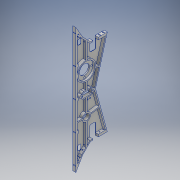
# Autodesk Inventor part: 옆판_왼쪽
Saved by Autodesk Inventor 2017 (Build 210142000, 142)
## iProperties
Part Number: 옆판_왼쪽
Material: 알루미늄 6061
Document SubType Name: Modeling
Designer: minom
Density: 2.7 g/cm^3
Appearance: 알루미늄 - 평지
Mass: 105.833 g
Surface Area: 460.964 cm^2
Volume: 39.1973 cm^3
Author: minom
Autodesk Inventor part; units mm, degrees
(part 1 of 2)
ref_plane "YZ Plane" through (0, 0, 0) normal (1, 0, 0) x (0, 1, 0)
ref_plane "XZ Plane" through (0, 0, 0) normal (0, 1, 0) x (-1, 0, 0)
ref_plane "XY Plane" through (0, 0, 0) normal (0, 0, 1) x (1, 0, 0)
sketch "스케치1" plane through (0, 0, 0) normal (1, 0, 0) x (0, 1, 0)
  line L0 (0, 0) -> (0, -320)
  line L1 (0, -320) -> (0, -270)
  line L2 (0, -270) -> (0, -290)
  line L3 (0, 0) -> (0, -50)
  line L4 (0, -50) -> (0, -30)
  line L5 (0, -30) -> (60, -30)
  line L6 (80, -50) -> (80, -270)
  line L7 (80, -270) -> (0, -270)
  line L8 (0, -290) -> (80, -290)
  line L9 (0, -50) -> (80, -50)
  line L10 (0, 0) -> (17.3205, -30)
  line L11 (0, 0) -> (34.641, 0) construction
  line L12 (17.3205, -30) -> (37.3205, -50)
  line L13 (17.3205, -30) -> (45.6048, -30) construction
  line L14 (0, -320) -> (17.3205, -290)
  line L15 (0, -320) -> (34.641, -320) construction
  line L16 (17.3205, -290) -> (37.3205, -270)
  line L17 (17.3205, -290) -> (45.6048, -290) construction
  dimension "d0" = 320
  dimension "d1" = 50
  dimension "d2" = 50
  dimension "d3" = 20
  dimension "d4" = 60
  dimension "d5" = 60
  dimension "d6" = 45
  dimension "d7" = 60
  dimension "d8" = 45
  dimension "d37" = 80
  constraints: 36 end point, 9 point on line, 4 equal length, 4 horizontal, 4 perpendicular, 1 parallel, 1 vertical
  measures "d0" distance of L0.start L0.end
  measures "d1" distance of L0.end L1.end
  measures "d2" distance of L0.start L3.end
  measures "d3" distance of L3.end L4.end
  measures "d4" distance of L4.end L5.end
  measures "d5" angle of L10 L11
  measures "d6" angle of L12 L13
  measures "d7" angle of L15 L14
  measures "d8" angle of L17 L16
  measures "d37" distance between parallel lines of L0 L6
extrude "돌출1" add sketch "스케치1" along normal blind 8
sketch "스케치2" plane through (8, 0, 0) normal (1, 0, 0) x (0, 0, -1)
  line L0 (270, 37.3205) -> (270, 80) projected
  line L1 (270, 80) -> (50, 80) projected
  line L2 (109, 80) -> (109, 27)
  circle A0 centre (109, 27) radius 21.25
  line L3 (50, 80) -> (50, 37.3205) projected
  line L4 (0, 0) -> (320, 0) projected
  dimension "d13" = 42.5
  dimension "d16" = 59
  dimension "d149" = 27
  constraints: 2 end point, 1 centre point, 1 coincident, 1 point on line
  measures "d13" diameter of A0
  measures "d16" distance between parallel lines of L2 L3
  measures "d149" distance from line of L4 L2.end
extrude "돌출2" cut sketch "스케치2" against normal blind 5
sketch "스케치3" plane through (3, 27, -109) normal (1, 0, 0) x (0, 0, -1)
  circle A0 centre (0, 0) radius 21.25 projected
  line L0 (-59, 10.3205) -> (-79, -9.6795) projected
  line L1 (-79, -9.6795) -> (-109, -27) projected
  line L2 (-109, -27) -> (211, -27) projected
  line L3 (211, -27) -> (181, -9.6795) projected
  line L4 (181, -9.6795) -> (161, 10.3205) projected
  line L5 (161, 10.3205) -> (161, 53) projected
  line L6 (161, 53) -> (-59, 53) projected
  line L7 (-59, 53) -> (-59, 10.3205) projected
  line L8 (0, 0) -> (0, 17.6)
  line L9 (0, 17.6) -> (0, -17.6)
  line L10 (0, 0) -> (17.6, 0)
  line L11 (17.6, 0) -> (-17.6, 0)
  circle A1 centre (-17.6, 0) radius 2.1
  circle A2 centre (0, 17.6) radius 2.1
  circle A3 centre (17.6, 0) radius 2.1
  circle A4 centre (0, -17.6) radius 2.1
  circle A5 centre (0, 0) radius 12.6
  dimension "d17" = 17.6
  dimension "d18" = 35.2
  dimension "d19" = 17.6
  dimension "d20" = 35.2
  dimension "d21" = 4.2
  dimension "d22" = 4.2
  dimension "d23" = 4.2
  dimension "d24" = 4.2
  dimension "d25" = 25.2
  constraints: 8 end point, 5 centre point, 5 coincident, 2 point on line, 1 horizontal, 1 vertical
  measures "d17" distance of L8.start L8.end
  measures "d18" distance of L8.end L9.end
  measures "d19" distance of L8.start L10.end
  measures "d20" distance of L10.end L11.end
  measures "d21" diameter of A1
  measures "d22" diameter of A2
  measures "d23" diameter of A3
  measures "d24" diameter of A4
  measures "d25" diameter of A5
extrude "돌출3" cut sketch "스케치3" against normal blind 3 contours L11 A5 L8 | L10 A5 L9 | L8 A5 L10 | L9 A5 L11 | A2 | A3 | A4 | A1
sketch "스케치4" plane through (0, 0, 0) normal (-1, 0, 0) x (0, 0, 1)
  line L0 (0, 0) -> (-320, 0) projected
  line L1 (-30, 17.3205) -> (0, 0) projected
  line L2 (-50, 37.3205) -> (-30, 17.3205) projected
  line L3 (-50, 80) -> (-50, 37.3205) projected
  line L4 (-270, 80) -> (-50, 80) projected
  line L5 (-270, 37.3205) -> (-270, 80) projected
  line L6 (-290, 17.3205) -> (-270, 37.3205) projected
  line L7 (-320, 0) -> (-290, 17.3205) projected
  line L8 (-50, 37.3205) -> (-50, 20.3205)
  line L9 (-290, 17.3205) -> (-270, 37.3205) projected
  line L10 (-270, 37.3205) -> (-270, 20.3205)
  line L11 (-48, 20.3205) -> (-39, 20.3205)
  line L12 (-37, 18.3205) -> (-37, 14.3205)
  line L13 (-39, 12.3205) -> (-48, 12.3205)
  line L14 (-50, 14.3205) -> (-50, 18.3205)
  line L15 (-272, 20.3205) -> (-281, 20.3205)
  line L16 (-283, 18.3205) -> (-283, 14.3205)
  line L17 (-281, 12.3205) -> (-272, 12.3205)
  line L18 (-270, 14.3205) -> (-270, 18.3205)
  arc A0 (-270, 18.3205) -> (-272, 20.3205) centre (-272, 18.3205) ccw
  arc A1 (-272, 12.3205) -> (-270, 14.3205) centre (-272, 14.3205) ccw
  arc A2 (-283, 14.3205) -> (-281, 12.3205) centre (-281, 14.3205) ccw
  arc A3 (-281, 20.3205) -> (-283, 18.3205) centre (-281, 18.3205) ccw
  arc A4 (-37, 18.3205) -> (-39, 20.3205) centre (-39, 18.3205) ccw
  arc A5 (-39, 12.3205) -> (-37, 14.3205) centre (-39, 14.3205) ccw
  arc A6 (-50, 14.3205) -> (-48, 12.3205) centre (-48, 14.3205) ccw
  arc A7 (-48, 20.3205) -> (-50, 18.3205) centre (-48, 18.3205) ccw
  point P0 (-37, 12.3205)
  point P1 (-37, 20.3205)
  point P2 (-50, 12.3205)
  point P3 (-283, 12.3205)
  point P4 (-283, 20.3205)
  point P5 (-270, 12.3205)
  dimension "d28" = 17
  dimension "d29" = 17
  dimension "d30" = 13
  dimension "d31" = 8
  dimension "d32" = 13
  dimension "d33" = 8
  dimension "d34" = 2
  constraints: 20 end point, 16 point on circle, 16 point on line, 16 tangent, 8 centre point, 7 equal radius, 4 parallel, 2 horizontal, 2 perpendicular, 2 vertical
  measures "d28" distance of L2.start L8.end
  measures "d29" distance of L5.start L10.end
  measures "d30" distance of point (-37, 12.321) point (-50, 12.321)
  measures "d31" distance of point (-37, 20.321) point (-37, 12.321)
  measures "d32" distance of point (-270, 12.321) point (-283, 12.321)
  measures "d33" distance of point (-283, 12.321) point (-283, 20.321)
  measures "d34" radius of A0
extrude "돌출4" cut sketch "스케치4" against normal blind 10 contours L11 A4 L12 A5 L13 A6 L14 A7 | A0 L18 A1 L17 A2 L16 A3 L15
sketch "스케치5" plane through (8, 0, 0) normal (1, 0, 0) x (0, 0, -1)
  arc A0 (272, 20.3205) -> (270, 18.3205) centre (272, 18.3205) ccw projected
  line L0 (272, 20.3205) -> (281, 20.3205) projected
  arc A1 (283, 18.3205) -> (281, 20.3205) centre (281, 18.3205) ccw projected
  line L1 (283, 18.3205) -> (283, 14.3205) projected
  arc A2 (281, 12.3205) -> (283, 14.3205) centre (281, 14.3205) ccw projected
  line L2 (281, 12.3205) -> (272, 12.3205) projected
  arc A3 (270, 14.3205) -> (272, 12.3205) centre (272, 14.3205) ccw projected
  line L3 (270, 14.3205) -> (270, 18.3205) projected
  arc A4 (39, 20.3205) -> (37, 18.3205) centre (39, 18.3205) ccw projected
  line L4 (39, 20.3205) -> (48, 20.3205) projected
  arc A5 (50, 18.3205) -> (48, 20.3205) centre (48, 18.3205) ccw projected
  line L5 (50, 18.3205) -> (50, 14.3205) projected
  arc A6 (48, 12.3205) -> (50, 14.3205) centre (48, 14.3205) ccw projected
  line L6 (48, 12.3205) -> (39, 12.3205) projected
  arc A7 (37, 14.3205) -> (39, 12.3205) centre (39, 14.3205) ccw projected
  line L7 (37, 14.3205) -> (37, 18.3205) projected
  circle A8 centre (109, 27) radius 21.25 projected
  line L8 (50, 37.3205) -> (30, 17.3205) projected
  line L9 (30, 17.3205) -> (0, 0) projected
  line L10 (0, 0) -> (320, 0) projected
  line L11 (320, 0) -> (290, 17.3205) projected
  line L12 (290, 17.3205) -> (270, 37.3205) projected
  line L13 (270, 37.3205) -> (270, 80) projected
  line L14 (270, 80) -> (50, 80) projected
  line L15 (50, 80) -> (50, 37.3205) projected
  circle A9 centre (211, 27) radius 7.55
  dimension "d38" = 15.1
  dimension "d39" = 102
  dimension "d150" = 27
  constraints: 1 centre point
  measures "d38" diameter of A9
  measures "d39" distance of A9.centre A8.centre
  measures "d150" distance from line of L10 A9.centre
extrude "돌출5" cut sketch "스케치5" against normal blind 10 contours A9
sketch "스케치6" plane through (0, 0, 0) normal (-1, 0, 0) x (0, 0, 1)
  circle A0 centre (-211, 27) radius 7.55 projected
  arc A1 (-270, 18.3205) -> (-272, 20.3205) centre (-272, 18.3205) ccw projected
  line L0 (-270, 18.3205) -> (-270, 14.3205) projected
  arc A2 (-272, 12.3205) -> (-270, 14.3205) centre (-272, 14.3205) ccw projected
  line L1 (-272, 12.3205) -> (-281, 12.3205) projected
  arc A3 (-283, 14.3205) -> (-281, 12.3205) centre (-281, 14.3205) ccw projected
  line L2 (-283, 14.3205) -> (-283, 18.3205) projected
  arc A4 (-281, 20.3205) -> (-283, 18.3205) centre (-281, 18.3205) ccw projected
  line L3 (-281, 20.3205) -> (-272, 20.3205) projected
  arc A5 (-37, 18.3205) -> (-39, 20.3205) centre (-39, 18.3205) ccw projected
  line L4 (-37, 18.3205) -> (-37, 14.3205) projected
  arc A6 (-39, 12.3205) -> (-37, 14.3205) centre (-39, 14.3205) ccw projected
  line L5 (-39, 12.3205) -> (-48, 12.3205) projected
  arc A7 (-50, 14.3205) -> (-48, 12.3205) centre (-48, 14.3205) ccw projected
  line L6 (-50, 14.3205) -> (-50, 18.3205) projected
  arc A8 (-48, 20.3205) -> (-50, 18.3205) centre (-48, 18.3205) ccw projected
  line L7 (-48, 20.3205) -> (-39, 20.3205) projected
  circle A9 centre (-109, 9.4) radius 2.1 projected
  circle A10 centre (-109, 44.6) radius 2.1 projected
  circle A11 centre (-91.4, 27) radius 2.1 projected
  circle A12 centre (-126.6, 27) radius 2.1 projected
  circle A13 centre (-109, 27) radius 12.6 projected
  line L8 (0, 0) -> (-320, 0) projected
  line L9 (-30, 17.3205) -> (0, 0) projected
  line L10 (-50, 37.3205) -> (-30, 17.3205) projected
  line L11 (-50, 80) -> (-50, 37.3205) projected
  line L12 (-270, 80) -> (-50, 80) projected
  line L13 (-270, 37.3205) -> (-270, 80) projected
  line L14 (-290, 17.3205) -> (-270, 37.3205) projected
  line L15 (-320, 0) -> (-290, 17.3205) projected
  line L16 (-164, 40) -> (-156, 40)
  line L17 (-154, 38) -> (-154, 20)
  line L18 (-156, 18) -> (-164, 18)
  line L19 (-166, 20) -> (-166, 38)
  arc A14 (-154, 38) -> (-156, 40) centre (-156, 38) ccw
  arc A15 (-156, 18) -> (-154, 20) centre (-156, 20) ccw
  arc A16 (-166, 20) -> (-164, 18) centre (-164, 20) ccw
  arc A17 (-164, 40) -> (-166, 38) centre (-164, 38) ccw
  point P0 (-154, 18)
  point P1 (-154, 40)
  point P2 (-166, 18)
  dimension "d42" = 12
  dimension "d43" = 22
  dimension "d44" = 40
  dimension "d45" = 104
  dimension "d46" = 2
  constraints: 8 end point, 8 point on circle, 8 tangent, 6 point on line, 4 centre point, 3 equal radius, 2 parallel, 1 horizontal, 1 perpendicular
  measures "d42" distance of point (-154, 18) point (-166, 18)
  measures "d43" distance of point (-154, 40) point (-154, 18)
  measures "d44" distance between parallel lines of L16 L12
  measures "d45" distance between parallel lines of L19 L13
  measures "d46" radius of A14
extrude "돌출6" cut sketch "스케치6" against normal blind 10 contours L16 A14 L17 A15 L18 A16 L19 A17
sketch "스케치8" plane through (8, 0, 0) normal (1, 0, 0) x (0, 0, -1)
  arc A0 (156, 40) -> (154, 38) centre (156, 38) ccw projected
  line L0 (156, 40) -> (164, 40) projected
  arc A1 (166, 38) -> (164, 40) centre (164, 38) ccw projected
  line L1 (166, 38) -> (166, 20) projected
  arc A2 (164, 18) -> (166, 20) centre (164, 20) ccw projected
  line L2 (164, 18) -> (156, 18) projected
  arc A3 (154, 20) -> (156, 18) centre (156, 20) ccw projected
  line L3 (154, 20) -> (154, 38) projected
  circle A4 centre (211, 27) radius 7.55 projected
  arc A5 (272, 20.3205) -> (270, 18.3205) centre (272, 18.3205) ccw projected
  line L4 (272, 20.3205) -> (281, 20.3205) projected
  arc A6 (283, 18.3205) -> (281, 20.3205) centre (281, 18.3205) ccw projected
  line L5 (283, 18.3205) -> (283, 14.3205) projected
  arc A7 (281, 12.3205) -> (283, 14.3205) centre (281, 14.3205) ccw projected
  line L6 (281, 12.3205) -> (272, 12.3205) projected
  arc A8 (270, 14.3205) -> (272, 12.3205) centre (272, 14.3205) ccw projected
  line L7 (270, 14.3205) -> (270, 18.3205) projected
  arc A9 (39, 20.3205) -> (37, 18.3205) centre (39, 18.3205) ccw projected
  line L8 (39, 20.3205) -> (48, 20.3205) projected
  arc A10 (50, 18.3205) -> (48, 20.3205) centre (48, 18.3205) ccw projected
  line L9 (50, 18.3205) -> (50, 14.3205) projected
  arc A11 (48, 12.3205) -> (50, 14.3205) centre (48, 14.3205) ccw projected
  line L10 (48, 12.3205) -> (39, 12.3205) projected
  arc A12 (37, 14.3205) -> (39, 12.3205) centre (39, 14.3205) ccw projected
  line L11 (37, 14.3205) -> (37, 18.3205) projected
  circle A13 centre (109, 27) radius 21.25 projected
  line L12 (50, 37.3205) -> (30, 17.3205) projected
  line L13 (30, 17.3205) -> (0, 0) projected
  line L14 (0, 0) -> (320, 0) projected
  line L15 (320, 0) -> (290, 17.3205) projected
  line L16 (290, 17.3205) -> (270, 37.3205) projected
  line L17 (270, 37.3205) -> (270, 80) projected
  line L18 (270, 80) -> (50, 80) projected
  line L19 (50, 80) -> (50, 37.3205) projected
  circle A14 centre (160, 43.5) radius 1.5
  circle A15 centre (160, 14.5) radius 1.5
  dimension "d61" = 3
  dimension "d62" = 3
  dimension "d63" = 3.5
  dimension "d64" = 6
  dimension "d65" = 3.5
  dimension "d66" = 6
  constraints: 2 centre point
  measures "d61" diameter of A14
  measures "d62" diameter of A15
  measures "d63" distance from line of L0 A14.centre
  measures "d64" distance from line of L3 A14.centre
  measures "d65" distance from line of L2 A15.centre
  measures "d66" distance from line of L1 A15.centre
extrude "돌출8" cut sketch "스케치8" against normal blind 10 contours A14 | A15
sketch "스케치9" plane through (0, 0, 0) normal (-1, 0, 0) x (0, 0, 1)
  circle A0 centre (-160, 43.5) radius 1.5 projected
  circle A1 centre (-160, 14.5) radius 1.5 projected
  arc A2 (-154, 38) -> (-156, 40) centre (-156, 38) ccw projected
  line L0 (-154, 38) -> (-154, 20) projected
  arc A3 (-156, 18) -> (-154, 20) centre (-156, 20) ccw projected
  line L1 (-156, 18) -> (-164, 18) projected
  arc A4 (-166, 20) -> (-164, 18) centre (-164, 20) ccw projected
  line L2 (-166, 20) -> (-166, 38) projected
  arc A5 (-164, 40) -> (-166, 38) centre (-164, 38) ccw projected
  line L3 (-164, 40) -> (-156, 40) projected
  circle A6 centre (-211, 27) radius 7.55 projected
  arc A7 (-270, 18.3205) -> (-272, 20.3205) centre (-272, 18.3205) ccw projected
  line L4 (-270, 18.3205) -> (-270, 14.3205) projected
  arc A8 (-272, 12.3205) -> (-270, 14.3205) centre (-272, 14.3205) ccw projected
  line L5 (-272, 12.3205) -> (-281, 12.3205) projected
  arc A9 (-283, 14.3205) -> (-281, 12.3205) centre (-281, 14.3205) ccw projected
  line L6 (-283, 14.3205) -> (-283, 18.3205) projected
  arc A10 (-281, 20.3205) -> (-283, 18.3205) centre (-281, 18.3205) ccw projected
  line L7 (-281, 20.3205) -> (-272, 20.3205) projected
  arc A11 (-37, 18.3205) -> (-39, 20.3205) centre (-39, 18.3205) ccw projected
  line L8 (-37, 18.3205) -> (-37, 14.3205) projected
  arc A12 (-39, 12.3205) -> (-37, 14.3205) centre (-39, 14.3205) ccw projected
  line L9 (-39, 12.3205) -> (-48, 12.3205) projected
  arc A13 (-50, 14.3205) -> (-48, 12.3205) centre (-48, 14.3205) ccw projected
  line L10 (-50, 14.3205) -> (-50, 18.3205) projected
  arc A14 (-48, 20.3205) -> (-50, 18.3205) centre (-48, 18.3205) ccw projected
  line L11 (-48, 20.3205) -> (-39, 20.3205) projected
  circle A15 centre (-109, 9.4) radius 2.1 projected
  circle A16 centre (-109, 44.6) radius 2.1 projected
  circle A17 centre (-91.4, 27) radius 2.1 projected
  circle A18 centre (-126.6, 27) radius 2.1 projected
  circle A19 centre (-109, 27) radius 12.6 projected
  line L12 (0, 0) -> (-320, 0) projected
  line L13 (-30, 17.3205) -> (0, 0) projected
  line L14 (-50, 37.3205) -> (-30, 17.3205) projected
  line L15 (-50, 80) -> (-50, 37.3205) projected
  line L16 (-270, 80) -> (-50, 80) projected
  line L17 (-270, 37.3205) -> (-270, 80) projected
  line L18 (-290, 17.3205) -> (-270, 37.3205) projected
  line L19 (-320, 0) -> (-290, 17.3205) projected
  line L20 (-50, 80) -> (-50, 37.3205) projected
  line L21 (-50, 57) -> (-78, 57)
  line L22 (-80, 55) -> (-80, 45)
  line L23 (-78, 43) -> (-50, 43)
  line L24 (-50, 43) -> (-50, 57)
  line L25 (-270, 37.3205) -> (-270, 80) projected
  line L26 (-270, 57) -> (-242, 57)
  line L27 (-240, 55) -> (-240, 45)
  line L28 (-242, 43) -> (-270, 43)
  line L29 (-270, 43) -> (-270, 57)
  arc A20 (-78, 57) -> (-80, 55) centre (-78, 55) ccw
  arc A21 (-80, 45) -> (-78, 43) centre (-78, 45) ccw
  arc A22 (-240, 55) -> (-242, 57) centre (-242, 55) ccw
  arc A23 (-242, 43) -> (-240, 45) centre (-242, 45) ccw
  point P0 (-80, 43)
  point P1 (-80, 57)
  point P2 (-240, 43)
  point P3 (-240, 57)
  dimension "d69" = 30
  dimension "d70" = 14
  dimension "d71" = 23
  dimension "d72" = 30
  dimension "d73" = 14
  dimension "d74" = 23
  dimension "d147" = 2
  constraints: 16 end point, 10 point on line, 8 point on circle, 8 tangent, 4 centre point, 4 parallel, 3 equal radius, 2 horizontal, 2 perpendicular
  measures "d69" distance of L23.end point (-80, 43)
  measures "d70" distance of point (-80, 43) point (-80, 57)
  measures "d71" distance between parallel lines of L21 L16
  measures "d72" distance of point (-240, 43) L28.end
  measures "d73" distance of point (-240, 57) point (-240, 43)
  measures "d74" distance between parallel lines of L26 L16
  measures "d147" radius of A20
extrude "돌출9" cut sketch "스케치9" against normal blind 10 contours L23 A21 L22 A20 L21 L15 | L17 L26 A22 L27 A23 L28
sketch "스케치18" plane through (8, 0, 0) normal (1, 0, 0) x (0, 0, -1)
  line L0 (50, 57) -> (78, 57) projected
  arc A0 (80, 55) -> (78, 57) centre (78, 55) ccw projected
  line L1 (80, 55) -> (80, 45) projected
  arc A1 (78, 43) -> (80, 45) centre (78, 45) ccw projected
  line L2 (78, 43) -> (50, 43) projected
  line L3 (50, 43) -> (50, 37.3205) projected
  line L4 (50, 37.3205) -> (30, 17.3205) projected
  line L5 (30, 17.3205) -> (0, 0) projected
  line L6 (0, 0) -> (320, 0) projected
  line L7 (320, 0) -> (290, 17.3205) projected
  line L8 (290, 17.3205) -> (270, 37.3205) projected
  line L9 (270, 37.3205) -> (270, 43) projected
  line L10 (270, 43) -> (242, 43) projected
  arc A2 (240, 45) -> (242, 43) centre (242, 45) ccw projected
  line L11 (240, 45) -> (240, 55) projected
  arc A3 (242, 57) -> (240, 55) centre (242, 55) ccw projected
  line L12 (242, 57) -> (270, 57) projected
  line L13 (270, 57) -> (270, 80) projected
  line L14 (270, 80) -> (50, 80) projected
  line L15 (50, 80) -> (50, 57) projected
  circle A4 centre (109, 27) radius 21.25 projected
  arc A5 (39, 20.3205) -> (37, 18.3205) centre (39, 18.3205) ccw projected
  line L16 (39, 20.3205) -> (48, 20.3205) projected
  arc A6 (50, 18.3205) -> (48, 20.3205) centre (48, 18.3205) ccw projected
  line L17 (50, 18.3205) -> (50, 14.3205) projected
  arc A7 (48, 12.3205) -> (50, 14.3205) centre (48, 14.3205) ccw projected
  line L18 (48, 12.3205) -> (39, 12.3205) projected
  arc A8 (37, 14.3205) -> (39, 12.3205) centre (39, 14.3205) ccw projected
  line L19 (37, 14.3205) -> (37, 18.3205) projected
  arc A9 (272, 20.3205) -> (270, 18.3205) centre (272, 18.3205) ccw projected
  line L20 (272, 20.3205) -> (281, 20.3205) projected
  arc A10 (283, 18.3205) -> (281, 20.3205) centre (281, 18.3205) ccw projected
  line L21 (283, 18.3205) -> (283, 14.3205) projected
  arc A11 (281, 12.3205) -> (283, 14.3205) centre (281, 14.3205) ccw projected
  line L22 (281, 12.3205) -> (272, 12.3205) projected
  arc A12 (270, 14.3205) -> (272, 12.3205) centre (272, 14.3205) ccw projected
  line L23 (270, 14.3205) -> (270, 18.3205) projected
  circle A13 centre (211, 27) radius 7.55 projected
  arc A14 (156, 40) -> (154, 38) centre (156, 38) ccw projected
  line L24 (156, 40) -> (164, 40) projected
  arc A15 (166, 38) -> (164, 40) centre (164, 38) ccw projected
  line L25 (166, 38) -> (166, 20) projected
  arc A16 (164, 18) -> (166, 20) centre (164, 20) ccw projected
  line L26 (164, 18) -> (156, 18) projected
  arc A17 (154, 20) -> (156, 18) centre (156, 20) ccw projected
  line L27 (154, 20) -> (154, 38) projected
  circle A18 centre (160, 14.5) radius 1.5 projected
  circle A19 centre (160, 43.5) radius 1.5 projected
  line L28 (50, 50) -> (270, 50)
  line L29 (0, 0) -> (320, 0) projected
  line L30 (160, 0) -> (160, 50)
  line L31 (270, 80) -> (50, 80) projected
  line L32 (270, 80) -> (160, 50)
  line L33 (50, 80) -> (160, 50)
  dimension "d148" = 50
  constraints: 8 end point, 2 midpoint, 1 parallel, 1 point on line
  measures "d148" distance between parallel lines of L6 L28
extrude "돌출18" cut sketch "스케치18" against normal blind 8 contours L14 L32 L33
sketch "스케치19" plane through (8, 0, 0) normal (1, 0, 0) x (0, 0, -1)
  circle A0 centre (160, 14.5) radius 1.5 projected
  arc A1 (156, 40) -> (154, 38) centre (156, 38) ccw projected
  line L0 (156, 40) -> (164, 40) projected
  arc A2 (166, 38) -> (164, 40) centre (164, 38) ccw projected
  line L1 (166, 38) -> (166, 20) projected
  arc A3 (164, 18) -> (166, 20) centre (164, 20) ccw projected
  line L2 (164, 18) -> (156, 18) projected
  arc A4 (154, 20) -> (156, 18) centre (156, 20) ccw projected
  line L3 (154, 20) -> (154, 38) projected
  circle A5 centre (211, 27) radius 7.55 projected
  arc A6 (272, 20.3205) -> (270, 18.3205) centre (272, 18.3205) ccw projected
  line L4 (272, 20.3205) -> (281, 20.3205) projected
  arc A7 (283, 18.3205) -> (281, 20.3205) centre (281, 18.3205) ccw projected
  line L5 (283, 18.3205) -> (283, 14.3205) projected
  arc A8 (281, 12.3205) -> (283, 14.3205) centre (281, 14.3205) ccw projected
  line L6 (281, 12.3205) -> (272, 12.3205) projected
  arc A9 (270, 14.3205) -> (272, 12.3205) centre (272, 14.3205) ccw projected
  line L7 (270, 14.3205) -> (270, 18.3205) projected
  arc A10 (39, 20.3205) -> (37, 18.3205) centre (39, 18.3205) ccw projected
  line L8 (39, 20.3205) -> (48, 20.3205) projected
  arc A11 (50, 18.3205) -> (48, 20.3205) centre (48, 18.3205) ccw projected
  line L9 (50, 18.3205) -> (50, 14.3205) projected
  arc A12 (48, 12.3205) -> (50, 14.3205) centre (48, 14.3205) ccw projected
  line L10 (48, 12.3205) -> (39, 12.3205) projected
  arc A13 (37, 14.3205) -> (39, 12.3205) centre (39, 14.3205) ccw projected
  line L11 (37, 14.3205) -> (37, 18.3205) projected
  circle A14 centre (109, 27) radius 21.25 projected
  line L12 (270, 80) -> (160, 50) projected
  line L13 (160, 50) -> (50, 80) projected
  line L14 (50, 80) -> (50, 57) projected
  line L15 (50, 57) -> (78, 57) projected
  arc A15 (80, 55) -> (78, 57) centre (78, 55) ccw projected
  line L16 (80, 55) -> (80, 45) projected
  arc A16 (78, 43) -> (80, 45) centre (78, 45) ccw projected
  line L17 (78, 43) -> (50, 43) projected
  line L18 (50, 43) -> (50, 37.3205) projected
  line L19 (50, 37.3205) -> (30, 17.3205) projected
  line L20 (30, 17.3205) -> (0, 0) projected
  line L21 (0, 0) -> (320, 0) projected
  line L22 (320, 0) -> (290, 17.3205) projected
  line L23 (290, 17.3205) -> (270, 37.3205) projected
  line L24 (270, 37.3205) -> (270, 43) projected
  line L25 (270, 43) -> (242, 43) projected
  arc A17 (240, 45) -> (242, 43) centre (242, 45) ccw projected
  line L26 (240, 45) -> (240, 55) projected
  arc A18 (242, 57) -> (240, 55) centre (242, 55) ccw projected
  line L27 (242, 57) -> (270, 57) projected
  line L28 (270, 57) -> (270, 80) projected
  line L29 (50, 80) -> (160, 50) projected
  line L30 (50, 37.3205) -> (30, 17.3205) projected
  line L31 (160, 50) -> (270, 80) projected
  line L32 (270, 80) -> (160, 50) projected
  line L33 (290, 17.3205) -> (270, 37.3205) projected
  line L34 (288.158, 14.9199) -> (308.8038, 3)
  line L35 (11.1962, 3) -> (31.842, 14.9199)
  line L36 (133.2036, 25.5) -> (150.9988, 25.5)
  line L37 (111.8539, 51.0815) -> (113.4025, 59.5988)
  line L38 (53, 36.0779) -> (53, 43)
  arc A19 (155.4309, 42.9675) -> (151, 38) centre (156, 38) ccw
  arc A20 (169, 38) -> (164.5691, 42.9675) centre (164, 38) ccw
  arc A21 (164.4697, 15.0209) -> (169.0012, 20) centre (164, 20) ccw
  arc A22 (150.9988, 20) -> (155.5303, 15.0209) centre (156, 20) ccw
  arc A23 (155.5303, 15.0209) -> (164.4697, 15.0209) centre (160, 14.5) ccw
  line L39 (267, 43) -> (267, 36.0779)
  line L40 (53, 36.0779) -> (45.4221, 28.5)
  line L41 (42.4221, 25.5) -> (31.842, 14.9199)
  line L42 (114.8055, 50.5448) -> (116.3076, 58.8065)
  line L43 (133.2036, 28.5) -> (151, 28.5)
  line L44 (84.7964, 28.5) -> (45.4221, 28.5)
  line L45 (84.7964, 25.5) -> (42.4221, 25.5)
  arc A24 (133.2036, 28.5) -> (114.8055, 50.5448) centre (109, 27) ccw
  line L46 (157.7403, 47.5067) -> (116.3076, 58.8065)
  arc A25 (111.8539, 51.0815) -> (84.7964, 28.5) centre (109, 27) ccw
  arc A26 (84.7964, 25.5) -> (105.5269, 3) centre (109, 27) ccw
  line L47 (105.5269, 3) -> (11.1962, 3)
  arc A27 (112.4731, 3) -> (133.2036, 25.5) centre (109, 27) ccw
  line L48 (113.4025, 59.5988) -> (53, 76.0722)
  line L49 (53, 57) -> (53, 76.0722)
  line L50 (150.9988, 20) -> (150.9988, 25.5)
  line L51 (151, 28.5) -> (151, 38)
  line L52 (169, 38) -> (169, 28.5)
  line L53 (169.0012, 25.5) -> (169.0012, 20)
  line L54 (207.6561, 37.006) -> (203.6898, 58.821)
  line L55 (210.6077, 37.5427) -> (206.5975, 59.5988)
  line L56 (221.4428, 25.5) -> (277.5779, 25.5)
  line L57 (212.5, 16.5572) -> (212.5, 3)
  line L58 (209.5, 16.5572) -> (209.5, 3)
  line L59 (200.5572, 25.5) -> (169.0012, 25.5)
  line L60 (200.5572, 28.5) -> (169, 28.5)
  line L61 (203.6898, 58.821) -> (162.2415, 47.5169)
  arc A28 (212.5, 16.5572) -> (221.4428, 25.5) centre (211, 27) ccw
  line L62 (308.8038, 3) -> (212.5, 3)
  line L63 (209.5, 3) -> (112.4731, 3)
  line L64 (221.4428, 28.5) -> (274.5779, 28.5)
  line L65 (288.158, 14.9199) -> (277.5779, 25.5)
  line L66 (274.5779, 28.5) -> (267, 36.0779)
  line L67 (267, 76.0722) -> (206.5975, 59.5988)
  line L68 (267, 76.0722) -> (267, 57)
  arc A29 (221.4428, 28.5) -> (210.6077, 37.5427) centre (211, 27) ccw
  arc A30 (207.6561, 37.006) -> (200.5572, 28.5) centre (211, 27) ccw
  arc A31 (200.5572, 25.5) -> (209.5, 16.5572) centre (211, 27) ccw
  circle A32 centre (160, 43.5) radius 1.5 projected
  arc A33 (157.7403, 47.5067) -> (155.4309, 42.9675) centre (160, 43.5) ccw
  arc A34 (164.5691, 42.9675) -> (162.2415, 47.5169) centre (160, 43.5) ccw
  dimension "d168" = 3
  dimension "d183" = 3
  dimension "d185" = 3
  dimension "d187" = 3
  dimension "d188" = 3
  dimension "d189" = 3
  dimension "d190" = 24.25
  dimension "d191" = 3
  dimension "d192" = 24.25
  dimension "d193" = 24.25
  dimension "d194" = 24.25
  dimension "d195" = 3
  dimension "d196" = 3
  dimension "d197" = 3
  dimension "d198" = 3
  dimension "d201" = 5
  dimension "d202" = 5
  dimension "d203" = 3
  dimension "d204" = 3
  dimension "d205" = 3
  dimension "d208" = 3
  dimension "d209" = 3
  dimension "d210" = 3
  dimension "d211" = 3
  constraints: 70 end point, 30 point on circle, 15 centre point, 8 parallel, 4 point on line
  measures "d168" radial gap between concentric circles of A0 A23
  measures "d183" distance between parallel lines of L14 L49
  measures "d185" distance between parallel lines of L13 L48
  measures "d187" distance between parallel lines of L18 L38
  measures "d188" distance between parallel lines of L19 L40
  measures "d189" distance between parallel lines of L45 L44
  measures "d190" radius of A25
  measures "d191" distance between parallel lines of L42 L37
  measures "d192" radius of A24
  measures "d193" radius of A27
  measures "d194" radius of A26
  measures "d195" distance between parallel lines of L21 L47
  measures "d196" distance between parallel lines of L21 L63
  measures "d197" distance between parallel lines of L43 L36
  measures "d198" distance between parallel lines of L3 L51
  measures "d201" radius of A20
  measures "d202" radius of A19
  measures "d203" distance between parallel lines of L13 L46
  measures "d204" distance between parallel lines of L19 L41
  measures "d205" distance between parallel lines of L20 L35
  measures "d208" distance between parallel lines of L12 L67
  measures "d209" distance between parallel lines of L28 L68
  measures "d210" distance between parallel lines of L24 L39
  measures "d211" distance between parallel lines of L23 L66
extrude "돌출21" cut sketch "스케치19" against normal blind 7.3 contours L27 A18 L26 A17 L25 L39 L66 L64 A29 L55 L67 L68 | L49 L48 L37 A25 L44 L40 L38 L17 A16 L16 A15 L15 | L34 L62 L57 A28 L56 L65 | L35 L41 L45 A26 L47 | L36 L50 A22 A23 A21 L53 L59 A31 L58 L63 A27 | A19 L51 L43 A24 L42 L46 A33 | A20 A34 L61 L54 A30 L60 L52
sketch "스케치20" plane through (8, 0, 0) normal (1, 0, 0) x (0, 0, -1)
  line L0 (267, 43) -> (267, 36.0779) projected
  line L1 (267, 36.0779) -> (274.5779, 28.5) projected
  line L2 (274.5779, 28.5) -> (221.4428, 28.5) projected
  arc A0 (221.4428, 28.5) -> (210.6077, 37.5427) centre (211, 27) ccw projected
  line L3 (210.6077, 37.5427) -> (206.5975, 59.5988) projected
  line L4 (206.5975, 59.5988) -> (267, 76.0722) projected
  line L5 (267, 76.0722) -> (267, 57) projected
  line L6 (267, 57) -> (270, 57) projected
  line L7 (270, 57) -> (270, 80) projected
  line L8 (270, 80) -> (160, 50) projected
  line L9 (160, 50) -> (50, 80) projected
  line L10 (50, 80) -> (50, 57) projected
  line L11 (50, 57) -> (53, 57) projected
  line L12 (53, 57) -> (53, 76.0722) projected
  line L13 (53, 76.0722) -> (113.4025, 59.5988) projected
  line L14 (113.4025, 59.5988) -> (111.8539, 51.0815) projected
  arc A1 (111.8539, 51.0815) -> (84.7964, 28.5) centre (109, 27) ccw projected
  line L15 (84.7964, 28.5) -> (45.4221, 28.5) projected
  line L16 (45.4221, 28.5) -> (53, 36.0779) projected
  line L17 (53, 36.0779) -> (53, 43) projected
  line L18 (53, 43) -> (50, 43) projected
  line L19 (50, 43) -> (50, 37.3205) projected
  line L20 (50, 37.3205) -> (30, 17.3205) projected
  line L21 (30, 17.3205) -> (0, 0) projected
  line L22 (0, 0) -> (320, 0) projected
  line L23 (320, 0) -> (290, 17.3205) projected
  line L24 (290, 17.3205) -> (270, 37.3205) projected
  line L25 (270, 37.3205) -> (270, 43) projected
  line L26 (270, 43) -> (267, 43) projected
  circle A2 centre (109, 27) radius 21.25 projected
  circle A3 centre (211, 27) radius 7.55 projected
  arc A4 (156, 40) -> (154, 38) centre (156, 38) ccw projected
  line L27 (156, 40) -> (164, 40) projected
  arc A5 (166, 38) -> (164, 40) centre (164, 38) ccw projected
  line L28 (166, 38) -> (166, 20) projected
  arc A6 (164, 18) -> (166, 20) centre (164, 20) ccw projected
  line L29 (164, 18) -> (156, 18) projected
  arc A7 (154, 20) -> (156, 18) centre (156, 20) ccw projected
  line L30 (154, 20) -> (154, 38) projected
  circle A8 centre (160, 14.5) radius 1.5 projected
  circle A9 centre (160, 43.5) radius 1.5 projected
  line L31 (277.5779, 25.5) -> (288.158, 14.9199) projected
  line L32 (288.158, 14.9199) -> (308.8038, 3) projected
  line L33 (308.8038, 3) -> (212.5, 3) projected
  line L34 (212.5, 3) -> (212.5, 16.5572) projected
  arc A10 (212.5, 16.5572) -> (221.4428, 25.5) centre (211, 27) ccw projected
  line L35 (221.4428, 25.5) -> (277.5779, 25.5) projected
  line L36 (105.5269, 3) -> (11.1962, 3) projected
  line L37 (11.1962, 3) -> (31.842, 14.9199) projected
  line L38 (31.842, 14.9199) -> (42.4221, 25.5) projected
  line L39 (42.4221, 25.5) -> (84.7964, 25.5) projected
  arc A11 (84.7964, 25.5) -> (105.5269, 3) centre (109, 27) ccw projected
  arc A12 (133.2036, 28.5) -> (114.8055, 50.5448) centre (109, 27) ccw projected
  line L40 (114.8055, 50.5448) -> (116.3076, 58.8065) projected
  line L41 (116.3076, 58.8065) -> (157.7403, 47.5067) projected
  arc A13 (157.7403, 47.5067) -> (155.4309, 42.9675) centre (160, 43.5) ccw projected
  arc A14 (155.4309, 42.9675) -> (151, 38) centre (156, 38) ccw projected
  line L42 (151, 38) -> (151, 28.5) projected
  line L43 (151, 28.5) -> (133.2036, 28.5) projected
  line L44 (169, 28.5) -> (169, 38) projected
  arc A15 (169, 38) -> (164.5691, 42.9675) centre (164, 38) ccw projected
  arc A16 (164.5691, 42.9675) -> (162.2415, 47.5169) centre (160, 43.5) ccw projected
  line L45 (162.2415, 47.5169) -> (203.6898, 58.821) projected
  line L46 (203.6898, 58.821) -> (207.6561, 37.006) projected
  arc A17 (207.6561, 37.006) -> (200.5572, 28.5) centre (211, 27) ccw projected
  line L47 (200.5572, 28.5) -> (169, 28.5) projected
  arc A18 (112.4731, 3) -> (133.2036, 25.5) centre (109, 27) ccw projected
  line L48 (133.2036, 25.5) -> (150.9988, 25.5) projected
  line L49 (150.9988, 25.5) -> (150.9988, 20) projected
  arc A19 (150.9988, 20) -> (155.5303, 15.0209) centre (156, 20) ccw projected
  arc A20 (155.5303, 15.0209) -> (164.4697, 15.0209) centre (160, 14.5) ccw projected
  arc A21 (164.4697, 15.0209) -> (169.0012, 20) centre (164, 20) ccw projected
  line L50 (169.0012, 20) -> (169.0012, 25.5) projected
  line L51 (169.0012, 25.5) -> (200.5572, 25.5) projected
  arc A22 (200.5572, 25.5) -> (209.5, 16.5572) centre (211, 27) ccw projected
  line L52 (209.5, 16.5572) -> (209.5, 3) projected
  line L53 (209.5, 3) -> (112.4731, 3) projected
  line L54 (53, 57) -> (56, 57)
  line L55 (78, 57) -> (50, 57) projected
  line L56 (56, 57) -> (56, 75.2541)
  line L57 (267, 57) -> (264, 57)
  line L58 (264, 57) -> (264, 75.2541)
  line L59 (242, 43) -> (270, 43) projected
  line L60 (50, 43) -> (78, 43) projected
  line L61 (0, 0) -> (14, 0)
  line L62 (14, 0) -> (87, 0)
  line L63 (87, 0) -> (160, 0)
  line L64 (0, 0) -> (320, 0) projected
  line L65 (160, 0) -> (233, 0)
  line L66 (233, 0) -> (306, 0)
  line L67 (306, 0) -> (320, 0)
  line L68 (308.8038, 3) -> (302, 3)
  line L69 (302, 3) -> (302, 6.9282)
  line L70 (0, 0) -> (320, 0) projected
  line L71 (105.5269, 3) -> (11.1962, 3) projected
  line L72 (229, 6) -> (237, 6)
  line L73 (237, 6) -> (237, 3)
  line L74 (237, 3) -> (229, 3)
  line L75 (229, 3) -> (229, 6)
  line L76 (156, 3) -> (156, 6)
  line L77 (164, 3) -> (156, 3)
  line L78 (156, 6) -> (164, 6)
  line L79 (164, 6) -> (164, 3)
  line L80 (91, 3) -> (83, 3)
  line L81 (83, 6) -> (91, 6)
  line L82 (91, 6) -> (91, 3)
  line L83 (83, 3) -> (83, 6)
  line L84 (18, 3) -> (11.1962, 3)
  line L85 (18, 6.9282) -> (18, 3)
  line L86 (288.158, 14.9199) -> (308.8038, 3) projected
  line L87 (302, 6.9282) -> (308.8038, 3)
  line L88 (11.1962, 3) -> (31.842, 14.9199) projected
  line L89 (18, 6.9282) -> (11.1962, 3)
  line L90 (0, 0) -> (22.5383, 13.0125)
  line L91 (30, 17.3205) -> (0, 0) projected
  line L92 (22.5383, 13.0125) -> (24.0383, 10.4144)
  line L93 (320, 0) -> (297.4617, 13.0125)
  line L94 (320, 0) -> (290, 17.3205) projected
  line L95 (297.4617, 13.0125) -> (295.9617, 10.4144)
  line L96 (298.9928, 8.6644) -> (292.9306, 12.1644)
  line L97 (292.9306, 12.1644) -> (291.4306, 9.5663)
  line L98 (291.4306, 9.5663) -> (297.4928, 6.0663)
  line L99 (297.4928, 6.0663) -> (298.9928, 8.6644)
  line L100 (24.0383, 10.4144) -> (27.0694, 12.1644)
  line L101 (27.0694, 12.1644) -> (28.5694, 9.5663)
  line L102 (28.5694, 9.5663) -> (22.5072, 6.0663)
  line L103 (22.5072, 6.0663) -> (21.0072, 8.6644)
  line L104 (24.0383, 10.4144) -> (21.0072, 8.6644)
  dimension "d217" = 3
  dimension "d221" = 14
  dimension "d222" = 73
  dimension "d223" = 73
  dimension "d224" = 73
  dimension "d225" = 73
  dimension "d231" = 8
  dimension "d232" = 3
  dimension "d233" = 8
  dimension "d234" = 3
  dimension "d235" = 8
  dimension "d236" = 3
  dimension "d239" = 26.025
  dimension "d240" = 26.025
  dimension "d244" = 7
  dimension "d245" = 3
  dimension "d246" = 7
  dimension "d247" = 3.5
  dimension "d248" = 3
  dimension "d249" = 7
  constraints: 82 end point, 19 point on line, 12 perpendicular, 6 parallel, 4 collinear, 3 horizontal, 1 midpoint
  measures "d217" distance of L11.end L54.end
  measures "d221" distance of L21.end L61.end
  measures "d222" distance of L61.end L62.end
  measures "d223" distance of L62.end L63.end
  measures "d224" distance of L63.end L65.end
  measures "d225" distance of L65.end L66.end
  measures "d231" distance of L74.start L75.start
  measures "d232" distance of L72.end L74.start
  measures "d233" distance of L77.start L77.end
  measures "d234" distance of L78.end L77.start
  measures "d235" distance of L80.start L83.start
  measures "d236" distance of L81.end L80.start
  measures "d239" distance of L21.end L90.end
  measures "d240" distance of L22.end L93.end
  measures "d244" distance of L96.start L96.end
  measures "d245" distance of L96.end L97.end
  measures "d246" distance of L97.end L98.end
  measures "d247" distance of L92.end L100.end
  measures "d248" distance of L100.end L101.end
  measures "d249" distance of L101.end L102.end
extrude "돌출25" add sketch "스케치20" against normal blind 7.3 contours L37 L101 L102 L103 | L32 L99 L98 L97 | L4 L5 L57 L58 | L32 L33 L69 | L33 L75 L72 L73 | L12 L13 L56 L54 | L85 L36 L37 | L83 L81 L82 L36 | L76 L78 L79 L53
sketch "스케치7" plane through (0, 0, -320) normal (0, -1, 0) x (1, 0, 0)
  line L0 (0, 320) -> (0, 0) projected
  line L1 (0, 0) -> (8, 0) projected
  line L2 (8, 320) -> (8, 0) projected
  line L3 (0, 320) -> (8, 320) projected
  line L4 (4, 0) -> (4, 14)
  line L5 (4, 14) -> (4, 87)
  line L6 (4, 87) -> (4, 160)
  line L7 (4, 160) -> (4, 233)
  line L8 (4, 233) -> (4, 306)
  line L9 (4, 306) -> (4, 320)
  line L10 (0, 320) -> (8, 320) projected
  circle A0 centre (4, 306) radius 1.25
  circle A1 centre (4, 233) radius 1.25
  circle A2 centre (4, 160) radius 1.25
  circle A3 centre (4, 87) radius 1.25
  circle A4 centre (4, 14) radius 1.25
  dimension "d49" = 14
  dimension "d50" = 73
  dimension "d51" = 73
  dimension "d52" = 73
  dimension "d53" = 73
  dimension "d54" = 2.5
  dimension "d55" = 2.5
  dimension "d56" = 2.5
  dimension "d57" = 2.5
  dimension "d58" = 2.5
  constraints: 12 end point, 5 centre point, 5 coincident, 4 point on line, 2 midpoint, 1 vertical
  measures "d49" distance of L4.start L4.end
  measures "d50" distance of L4.end L5.end
  measures "d51" distance of L5.end L6.end
  measures "d52" distance of L6.end L7.end
  measures "d53" distance of L7.end L8.end
  measures "d54" diameter of A0
  measures "d55" diameter of A1
  measures "d56" diameter of A2
  measures "d57" diameter of A3
  measures "d58" diameter of A4
extrude "돌출7" cut sketch "스케치7" against normal blind 6.1 contours A0 L8 L9 | L9 L8 A0 | A4 L5 L4 | L4 L5 A4 | A1 L7 L8 | L8 L7 A1 | A3 L6 L5 | L5 L6 A3 | A2 L6 L7 | L7 L6 A2
sketch "스케치12" plane through (0, 17.3205, -30) normal (0, 0.7071, 0.7071) x (1, 0, 0)
  circle A0 centre (263.8, 8.0202) radius 1.6 projected
  circle A1 centre (223.8, 18.0202) radius 1.6 projected
  circle A2 centre (4, 18.0202) radius 1.6 projected
  circle A3 centre (-36, 18.0202) radius 1.6 projected
  circle A4 centre (-36, 8.0202) radius 1.6 projected
  circle A5 centre (4, 8.0202) radius 1.6 projected
  circle A6 centre (223.8, 8.0202) radius 1.6 projected
  circle A7 centre (263.8, 18.0202) radius 1.6 projected
  line L0 (-41.1, 27.0202) -> (268.9, 27.0202) projected
  line L1 (-41.1, 1.0202) -> (-41.1, 27.0202) projected
  line L2 (268.9, 1.0202) -> (121.9, 1.0202) projected
  line L3 (105.9, 1.0202) -> (-41.1, 1.0202) projected
  line L4 (268.9, 27.0202) -> (268.9, 1.0202) projected
  circle A8 centre (4, 18.0202) radius 1.25
  circle A9 centre (4, 8.0202) radius 1.25
  line L5 (105.9, 1.0202) -> (105.9, 8.0202) projected
  arc A10 (107.9, 10.0202) -> (105.9, 8.0202) centre (107.9, 8.0202) ccw projected
  line L6 (107.9, 10.0202) -> (119.9, 10.0202) projected
  arc A11 (121.9, 8.0202) -> (119.9, 10.0202) centre (119.9, 8.0202) ccw projected
  line L7 (121.9, 8.0202) -> (121.9, 1.0202) projected
  circle A12 centre (71, 18.0202) radius 1.6 projected
  circle A13 centre (156.8, 8.0202) radius 1.6 projected
  circle A14 centre (156.8, 18.0202) radius 1.6 projected
  circle A15 centre (71, 8.0202) radius 1.6 projected
  point P0 (0, -33.4607)
  dimension "d93" = 2.5
  dimension "d94" = 2.5
  constraints: 2 centre point, 2 coincident
  measures "d93" diameter of A8
  measures "d94" diameter of A9
extrude "돌출12" cut sketch "스케치12" against normal blind 6.1 contours A8 | A9
sketch "스케치15" plane through (8, 37.3205, -270) normal (0, 0.7071, -0.7071) x (-1, 0, 0)
  circle A0 centre (44, -20.2843) radius 1.6 projected
  circle A1 centre (4, -10.2843) radius 1.6 projected
  circle A2 centre (-215.8, -10.2843) radius 1.6 projected
  circle A3 centre (-255.8, -10.2843) radius 1.6 projected
  circle A4 centre (-255.8, -20.2843) radius 1.6 projected
  circle A5 centre (-215.8, -20.2843) radius 1.6 projected
  circle A6 centre (4, -20.2843) radius 1.6 projected
  circle A7 centre (44, -10.2843) radius 1.6 projected
  line L0 (-260.9, -1.2843) -> (49.1, -1.2843) projected
  line L1 (-260.9, -27.2843) -> (-260.9, -1.2843) projected
  line L2 (49.1, -27.2843) -> (-97.9, -27.2843) projected
  line L3 (-113.9, -27.2843) -> (-260.9, -27.2843) projected
  line L4 (49.1, -1.2843) -> (49.1, -27.2843) projected
  circle A8 centre (4, -10.2843) radius 1.25
  circle A9 centre (4, -20.2843) radius 1.25
  line L5 (-113.9, -27.2843) -> (-113.9, -20.2843) projected
  arc A10 (-111.9, -18.2843) -> (-113.9, -20.2843) centre (-111.9, -20.2843) ccw projected
  line L6 (-111.9, -18.2843) -> (-99.9, -18.2843) projected
  arc A11 (-97.9, -20.2843) -> (-99.9, -18.2843) centre (-99.9, -20.2843) ccw projected
  line L7 (-97.9, -20.2843) -> (-97.9, -27.2843) projected
  circle A12 centre (-148.8, -10.2843) radius 1.6 projected
  circle A13 centre (-63, -20.2843) radius 1.6 projected
  circle A14 centre (-63, -10.2843) radius 1.6 projected
  circle A15 centre (-148.8, -20.2843) radius 1.6 projected
  point P0 (8, 164.5292)
  dimension "d105" = 2.5
  dimension "d106" = 2.5
  constraints: 2 centre point, 2 coincident
  measures "d105" diameter of A8
  measures "d106" diameter of A9
extrude "돌출15" cut sketch "스케치15" against normal blind 6.1 contours A8 | A9
sketch "스케치21" plane through (0, 57, -50) normal (0, 0, 1) x (1, 0, 0)
  circle A0 centre (-36, 17) radius 1.5 projected
  circle A1 centre (4, 17) radius 1.5 projected
  circle A2 centre (223.8, 17) radius 1.5 projected
  circle A3 centre (263.8, 17) radius 1.5 projected
  circle A4 centre (263.8, 7) radius 1.5 projected
  circle A5 centre (223.8, 7) radius 1.5 projected
  circle A6 centre (4, 7) radius 1.5 projected
  circle A7 centre (-36, 7) radius 1.5 projected
  line L0 (153.9, -14) -> (73.9, -14) projected
  line L1 (73.9, -14) -> (73.9, 0) projected
  line L2 (73.9, 0) -> (153.9, 0) projected
  line L3 (153.9, 0) -> (153.9, -14) projected
  line L4 (38.9, 0) -> (38.9, -14) projected
  line L5 (38.9, -14) -> (-31.1, -14) projected
  line L6 (-31.1, -14) -> (-31.1, 0) projected
  line L7 (-31.1, 0) -> (38.9, 0) projected
  line L8 (258.9, -14) -> (188.9, -14) projected
  line L9 (188.9, -14) -> (188.9, 0) projected
  line L10 (188.9, 0) -> (258.9, 0) projected
  line L11 (258.9, 0) -> (258.9, -14) projected
  line L12 (268.9, 23) -> (268.9, -17) projected
  line L13 (-41.1, 23) -> (268.9, 23) projected
  line L14 (-41.1, -17) -> (-41.1, 23) projected
  line L15 (268.9, -17) -> (-41.1, -17) projected
  circle A8 centre (4, 17) radius 1.25
  circle A9 centre (4, 7) radius 1.25
  point P0 (0, -57)
  dimension "d252" = 2.5
  dimension "d253" = 2.5
  constraints: 2 centre point, 2 coincident
  measures "d252" diameter of A8
  measures "d253" diameter of A9
extrude "돌출23" cut sketch "스케치21" against normal blind 6.1 contours A1 | A6 | A8 | A9
sketch "스케치22" plane through (8, 57, -270) normal (0, 0, -1) x (-1, 0, 0)
  circle A0 centre (-255.8, 17) radius 1.5 projected
  circle A1 centre (-215.8, 17) radius 1.5 projected
  circle A2 centre (4, 17) radius 1.5 projected
  circle A3 centre (44, 17) radius 1.5 projected
  circle A4 centre (44, 7) radius 1.5 projected
  circle A5 centre (4, 7) radius 1.5 projected
  circle A6 centre (-215.8, 7) radius 1.5 projected
  circle A7 centre (-255.8, 7) radius 1.5 projected
  line L0 (-65.9, -14) -> (-145.9, -14) projected
  line L1 (-145.9, -14) -> (-145.9, 0) projected
  line L2 (-145.9, 0) -> (-65.9, 0) projected
  line L3 (-65.9, 0) -> (-65.9, -14) projected
  line L4 (-180.9, 0) -> (-180.9, -14) projected
  line L5 (-180.9, -14) -> (-250.9, -14) projected
  line L6 (-250.9, -14) -> (-250.9, 0) projected
  line L7 (-250.9, 0) -> (-180.9, 0) projected
  line L8 (39.1, -14) -> (-30.9, -14) projected
  line L9 (-30.9, -14) -> (-30.9, 0) projected
  line L10 (-30.9, 0) -> (39.1, 0) projected
  line L11 (39.1, 0) -> (39.1, -14) projected
  line L12 (49.1, 23) -> (49.1, -17) projected
  line L13 (-260.9, 23) -> (49.1, 23) projected
  line L14 (-260.9, -17) -> (-260.9, 23) projected
  line L15 (49.1, -17) -> (-260.9, -17) projected
  circle A8 centre (4, 17) radius 1.25
  circle A9 centre (4, 7) radius 1.25
  point P0 (8, -57)
  dimension "d256" = 2.5
  dimension "d257" = 2.5
  constraints: 2 centre point, 2 coincident
  measures "d256" diameter of A8
  measures "d257" diameter of A9
extrude "돌출24" cut sketch "스케치22" against normal blind 6.1 contours A2 | A8 | A9
sketch "스케치23" plane through (0, 17.3205, -290) normal (0, 0.866, -0.5) x (1, 0, 0)
  circle A0 centre (71, 19.1163) radius 1.5 projected
  circle A1 centre (156.8, 9.1163) radius 1.5 projected
  circle A2 centre (156.8, 19.1163) radius 1.5 projected
  circle A3 centre (71, 9.1163) radius 1.5 projected
  circle A4 centre (-36, 9.1163) radius 1.5 projected
  circle A5 centre (4, 19.1163) radius 1.5 projected
  circle A6 centre (223.8, 9.1163) radius 1.5 projected
  circle A7 centre (263.8, 9.1163) radius 1.5 projected
  circle A8 centre (263.8, 19.1163) radius 1.5 projected
  circle A9 centre (223.8, 19.1163) radius 1.5 projected
  circle A10 centre (4, 9.1163) radius 1.5 projected
  circle A11 centre (-36, 19.1163) radius 1.5 projected
  line L0 (105.9, 1.1163) -> (105.9, 8.1163) projected
  arc A12 (107.9, 10.1163) -> (105.9, 8.1163) centre (107.9, 8.1163) ccw projected
  line L1 (107.9, 10.1163) -> (119.9, 10.1163) projected
  arc A13 (121.9, 8.1163) -> (119.9, 10.1163) centre (119.9, 8.1163) ccw projected
  line L2 (121.9, 8.1163) -> (121.9, 1.1163) projected
  line L3 (268.9, 1.1163) -> (121.9, 1.1163) projected
  line L4 (268.9, 35.1163) -> (268.9, 1.1163) projected
  line L5 (-41.1, 35.1163) -> (268.9, 35.1163) projected
  line L6 (-41.1, 1.1163) -> (-41.1, 35.1163) projected
  line L7 (105.9, 1.1163) -> (-41.1, 1.1163) projected
  circle A14 centre (4, 9.1163) radius 1.25
  circle A15 centre (4, 19.1163) radius 1.25
  point P0 (0, -242.4871)
  dimension "d262" = 2.5
  dimension "d263" = 2.5
  constraints: 2 centre point, 2 coincident
  measures "d262" diameter of A14
  measures "d263" diameter of A15
extrude "돌출26" cut sketch "스케치23" against normal blind 6.1 contours A14 | A15
sketch "스케치24" plane through (0, 0, 0) normal (0, 0.866, 0.5) x (1, 0, 0)
  circle A0 centre (156.8, 15.5247) radius 1.5 projected
  circle A1 centre (71, 25.5247) radius 1.5 projected
  circle A2 centre (71, 15.5247) radius 1.5 projected
  circle A3 centre (156.8, 25.5247) radius 1.5 projected
  circle A4 centre (263.8, 25.5247) radius 1.5 projected
  circle A5 centre (223.8, 15.5247) radius 1.5 projected
  circle A6 centre (4, 25.5247) radius 1.5 projected
  circle A7 centre (-36, 25.5247) radius 1.5 projected
  circle A8 centre (-36, 15.5247) radius 1.5 projected
  circle A9 centre (4, 15.5247) radius 1.5 projected
  circle A10 centre (223.8, 25.5247) radius 1.5 projected
  circle A11 centre (263.8, 15.5247) radius 1.5 projected
  line L0 (121.9, 33.5247) -> (121.9, 26.5247) projected
  arc A12 (119.9, 24.5247) -> (121.9, 26.5247) centre (119.9, 26.5247) ccw projected
  line L1 (119.9, 24.5247) -> (107.9, 24.5247) projected
  arc A13 (105.9, 26.5247) -> (107.9, 24.5247) centre (107.9, 26.5247) ccw projected
  line L2 (105.9, 26.5247) -> (105.9, 33.5247) projected
  line L3 (-41.1, 33.5247) -> (105.9, 33.5247) projected
  line L4 (-41.1, -0.4753) -> (-41.1, 33.5247) projected
  line L5 (268.9, -0.4753) -> (-41.1, -0.4753) projected
  line L6 (268.9, 33.5247) -> (268.9, -0.4753) projected
  line L7 (121.9, 33.5247) -> (268.9, 33.5247) projected
  circle A14 centre (4, 25.5247) radius 1.25
  circle A15 centre (4, 15.5247) radius 1.25
  point P0 (0, 0)
  dimension "d266" = 2.5
  dimension "d267" = 2.5
  constraints: 2 centre point, 2 coincident
  measures "d266" diameter of A14
  measures "d267" diameter of A15
extrude "돌출27" cut sketch "스케치24" against normal blind 6.1 contours A14 | A15
sketch "스케치25" plane through (0, 0, 0) normal (-1, 0, 0) x (0, 0, 1)
  line L0 (-160, 50) -> (-270, 80) projected
  line L1 (-270, 57) -> (-270, 80) projected
  line L2 (-270, 57) -> (-242, 57) projected
  arc A0 (-240, 55) -> (-242, 57) centre (-242, 55) ccw projected
  line L3 (-240, 55) -> (-240, 45) projected
  arc A1 (-242, 43) -> (-240, 45) centre (-242, 45) ccw projected
  line L4 (-242, 43) -> (-270, 43) projected
  line L5 (-270, 37.3205) -> (-270, 43) projected
  line L6 (-290, 17.3205) -> (-270, 37.3205) projected
  line L7 (-320, 0) -> (-290, 17.3205) projected
  line L8 (0, 0) -> (-320, 0) projected
  line L9 (-30, 17.3205) -> (0, 0) projected
  line L10 (-50, 37.3205) -> (-30, 17.3205) projected
  line L11 (-50, 43) -> (-50, 37.3205) projected
  line L12 (-50, 43) -> (-78, 43) projected
  arc A2 (-80, 45) -> (-78, 43) centre (-78, 45) ccw projected
  line L13 (-80, 45) -> (-80, 55) projected
  arc A3 (-78, 57) -> (-80, 55) centre (-78, 55) ccw projected
  line L14 (-78, 57) -> (-50, 57) projected
  line L15 (-50, 80) -> (-50, 57) projected
  line L16 (-50, 80) -> (-160, 50) projected
  circle A4 centre (-160, 43.5) radius 1.5 projected
  circle A5 centre (-160, 14.5) radius 1.5 projected
  arc A6 (-154, 38) -> (-156, 40) centre (-156, 38) ccw projected
  line L17 (-154, 38) -> (-154, 20) projected
  arc A7 (-156, 18) -> (-154, 20) centre (-156, 20) ccw projected
  line L18 (-156, 18) -> (-164, 18) projected
  arc A8 (-166, 20) -> (-164, 18) centre (-164, 20) ccw projected
  line L19 (-166, 20) -> (-166, 38) projected
  arc A9 (-164, 40) -> (-166, 38) centre (-164, 38) ccw projected
  line L20 (-164, 40) -> (-156, 40) projected
  circle A10 centre (-211, 27) radius 7.55 projected
  arc A11 (-270, 18.3205) -> (-272, 20.3205) centre (-272, 18.3205) ccw projected
  line L21 (-270, 18.3205) -> (-270, 14.3205) projected
  arc A12 (-272, 12.3205) -> (-270, 14.3205) centre (-272, 14.3205) ccw projected
  line L22 (-272, 12.3205) -> (-281, 12.3205) projected
  arc A13 (-283, 14.3205) -> (-281, 12.3205) centre (-281, 14.3205) ccw projected
  line L23 (-283, 14.3205) -> (-283, 18.3205) projected
  arc A14 (-281, 20.3205) -> (-283, 18.3205) centre (-281, 18.3205) ccw projected
  line L24 (-281, 20.3205) -> (-272, 20.3205) projected
  arc A15 (-37, 18.3205) -> (-39, 20.3205) centre (-39, 18.3205) ccw projected
  line L25 (-37, 18.3205) -> (-37, 14.3205) projected
  arc A16 (-39, 12.3205) -> (-37, 14.3205) centre (-39, 14.3205) ccw projected
  line L26 (-39, 12.3205) -> (-48, 12.3205) projected
  arc A17 (-50, 14.3205) -> (-48, 12.3205) centre (-48, 14.3205) ccw projected
  line L27 (-50, 14.3205) -> (-50, 18.3205) projected
  arc A18 (-48, 20.3205) -> (-50, 18.3205) centre (-48, 18.3205) ccw projected
  line L28 (-48, 20.3205) -> (-39, 20.3205) projected
  circle A19 centre (-109, 9.4) radius 2.1 projected
  circle A20 centre (-109, 44.6) radius 2.1 projected
  circle A21 centre (-91.4, 27) radius 2.1 projected
  circle A22 centre (-126.6, 27) radius 2.1 projected
  circle A23 centre (-109, 27) radius 12.6 projected
  line L29 (0, 0) -> (-320, 0) projected
  line L30 (-181, 0) -> (-181, 43.5)
  circle A24 centre (-181, 43.5) radius 1.5
  circle A25 centre (-181, 37.5) radius 1.5
  circle A26 centre (-181, 31.5) radius 1.5
  dimension "d270" = 15
  dimension "d271" = 3
  dimension "d272" = 3
  dimension "d273" = 3
  dimension "d274" = 6
  dimension "d275" = 21
  dimension "d276" = 6
  constraints: 3 centre point, 3 point on line, 2 end point, 1 coincident, 1 perpendicular
  measures "d270" distance between parallel lines of L19 L30
  measures "d271" diameter of A24
  measures "d272" diameter of A25
  measures "d273" diameter of A26
  measures "d274" distance of A25.centre L30.end
  measures "d275" distance of A4.centre L30.end
  measures "d276" distance of A26.centre A25.centre
extrude "돌출28" cut sketch "스케치25" against normal blind 2 contours A24 | A25 L30 | L30 A25 | A26 L30 | L30 A26